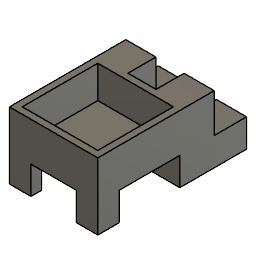
Pastillero (Autodesk Fusion 360 design; units mm, degrees)
Autodesk Fusion 360 part; units mm, degrees
sketch "Boceto1" plane through (0, 0, 0) normal (0, 1, 0) x (1, 0, 0)
  line L0 (-45, 25) -> (-4, 25)
  line L1 (-45, 25) -> (-45, -44)
  line L2 (-45, -44) -> (-4, -44)
  line L3 (-4, -44) -> (-4, 25)
  dimension "d1" = 41
  dimension "d2" = 69
  constraint horizontal L0
  constraint perpendicular L0 L1
  constraint perpendicular L1 L2
  constraint perpendicular L0 L3
  measures "d1" distance of L0.start L0.end
  measures "d2" distance of L0.start L1.end
extrude "Extruir1" add sketch "Boceto1" along normal blind 31
sketch "Boceto2" plane through (0, 31, 0) normal (0, 1, 0) x (-1, 0, 0)
  line L0 (45, -25) -> (45, 44)
  line L1 (45, 44) -> (4, 44)
  line L2 (4, 44) -> (4, -25)
  line L3 (4, -25) -> (45, -25)
  line L4 (42, 41) -> (42, 31.833)
  line L5 (42, 41) -> (7, 41)
  line L6 (7, 41) -> (7, 6)
  line L7 (7, 6) -> (42, 6)
  line L8 (42, 6) -> (42, 31.833)
  dimension "d7" = 35
  dimension "d8" = 35
  constraint perpendicular L4 L5
  constraint perpendicular L5 L6
  constraint perpendicular L6 L7
  constraint perpendicular L7 L8
  measures "d7" distance of L4.start L5.end
  measures "d8" distance of L5.end L6.end
extrude "Extruir2" cut sketch "Boceto2" against normal blind 15 contours L4 L5 L6 L7 L8
sketch "Boceto3" plane through (0, 0, 44) normal (0, 0, 1) x (1, 0, 0)
  line L0 (-45, 0) -> (-4, 0)
  line L1 (-4, 0) -> (-4, 31)
  line L2 (-4, 31) -> (-45, 31)
  line L3 (-45, 31) -> (-45, 0)
  line L4 (-45, 0) -> (-45, 13)
  line L5 (-45, 13) -> (-4, 13)
  line L6 (-4, 13) -> (-4, 0)
  dimension "d11" = 13
  constraint coincident L0.start L3.end
  constraint perpendicular L0 L4
  constraint coincident L1 L5.end
  constraint perpendicular L1 L5
  constraint coincident L0.end L1.start
  measures "d11" distance of L0.start L4.end
extrude "Extruir3" cut sketch "Boceto3" against normal blind 38 contours L0 L1 L3 L4 L5 L6
sketch "Boceto4" plane through (0, 31, 0) normal (0, 1, 0) x (-1, 0, 0)
  line L0 (7, 6) -> (7, 41)
  line L1 (7, 41) -> (42, 41)
  line L2 (42, 41) -> (42, 6)
  line L3 (42, 6) -> (7, 6)
  line L4 (45, -25) -> (45, 44)
  line L5 (45, 44) -> (4, 44)
  line L6 (4, 44) -> (4, -25)
  line L7 (4, -25) -> (45, -25)
  line L8 (31, -25) -> (18, -25)
  line L9 (31, -25) -> (31, 3)
  line L10 (31, 3) -> (18, 3)
  line L11 (18, 3) -> (18, -25)
  dimension "d14" = 14
  dimension "d15" = 13
  dimension "d16" = 28
  constraint parallel L7 L8
  constraint perpendicular L9 L10
  constraint perpendicular L8 L11
  measures "d14" distance of L4.start L8.start
  measures "d15" distance of L8.start L8.end
  measures "d16" distance of L8.start L9.end
extrude "Extruir4" cut sketch "Boceto4" against normal blind 28 contours L7 L8 L9 L10 L11
sketch "Boceto5" plane through (-45, 0, 0) normal (-1, 0, 0) x (0, 0, 1)
  line L0 (6, 0) -> (6, 13)
  line L1 (6, 13) -> (44, 13)
  line L2 (44, 13) -> (44, 31)
  line L3 (44, 31) -> (-25, 31)
  line L4 (-25, 31) -> (-25, 0)
  line L5 (-25, 0) -> (6, 0)
  line L6 (-25, 31) -> (-10, 31)
  line L7 (-10, 31) -> (-10, 13)
  line L8 (-10, 13) -> (-25, 13)
  line L9 (-25, 13) -> (-25, 31)
  dimension "d19" = 15
  dimension "d20" = 18
  constraint coincident L3.end L4.start
  constraint perpendicular L4 L6
  constraint perpendicular L6 L7
  constraint coincident L4 L8.end
  constraint perpendicular L4 L8
  measures "d19" distance of L3.end L6.end
  measures "d20" distance of L6.end L7.end
extrude "Extruir5" cut sketch "Boceto5" against normal blind 50 contours L3 L4 L6 L7 L8 L9
sketch "Boceto6" plane through (0, 0, 6) normal (0, 0, 1) x (1, 0, 0)
  line L0 (-45, 0) -> (-4, 0)
  line L1 (-4, 0) -> (-4, 13)
  line L2 (-4, 13) -> (-45, 13)
  line L3 (-45, 13) -> (-45, 0)
  line L4 (-31, 13) -> (-18, 13)
  line L5 (-18, 13) -> (-18, 3)
  line L6 (-18, 3) -> (-31, 3)
  line L7 (-31, 3) -> (-31, 13)
  dimension "d23" = 14
  dimension "d24" = 13
  dimension "d25" = 10
  constraint parallel L2 L4
  constraint perpendicular L4 L5
  constraint perpendicular L5 L6
  constraint perpendicular L4 L7
  measures "d23" distance of L2.end L4.start
  measures "d24" distance of L4.start L4.end
  measures "d25" distance of L4.end L5.end
extrude "Extruir6" cut sketch "Boceto6" against normal blind 30 contours L2 L4 L5 L6 L7
sketch "Boceto7" plane through (0, 0, 3) normal (0, 0, -1) x (-1, 0, 0)
  line L0 (18, 13) -> (31, 13)
  line L1 (31, 13) -> (31, 31)
  line L2 (31, 31) -> (18, 31)
  line L3 (18, 31) -> (18, 13)
  line L4 (18, 13) -> (31, 13)
  line L5 (31, 13) -> (31, 22.5)
  line L6 (31, 22.5) -> (18, 22.5)
  line L7 (18, 22.5) -> (18, 13)
  dimension "d28" = 9.5
  constraint coincident L0.start L3.end
  constraint coincident L0.end L1.start
  constraint perpendicular L4 L5
  constraint coincident L3 L6.end
  constraint perpendicular L3 L6
  measures "d28" distance of L0.end L5.end
extrude "Extruir7" add sketch "Boceto7" along normal blind 4.5 contours L0 L1 L3 L4 L5 L6 L7
sketch "Boceto8" plane through (0, 13, 0) normal (0, -1, 0) x (1, 0, 0)
  line L0 (-4, 44) -> (-45, 44)
  line L1 (-45, 44) -> (-45, 6)
  line L2 (-45, 6) -> (-31, 6)
  line L3 (-31, 6) -> (-31, -1.5)
  line L4 (-31, -1.5) -> (-18, -1.5)
  line L5 (-18, -1.5) -> (-18, 6)
  line L6 (-18, 6) -> (-4, 6)
  line L7 (-4, 6) -> (-4, 44)
  line L8 (-45, 44) -> (-35, 44)
  line L9 (-35, 44) -> (-35, 34)
  line L10 (-35, 34) -> (-45, 34)
  line L11 (-45, 34) -> (-45, 44)
  line L12 (-4, 44) -> (-14, 44)
  line L13 (-14, 44) -> (-14, 34)
  line L14 (-14, 34) -> (-4, 34)
  line L15 (-4, 34) -> (-4, 44)
  constraint horizontal L8
  constraint vertical L9
  constraint horizontal L10
  constraint vertical L11
  constraint coincident L0.end L1.start
  constraint horizontal L12
  constraint vertical L13
  constraint horizontal L14
  constraint vertical L15
  constraint coincident L0.start L7.end
extrude "Extruir8" add sketch "Boceto8" along normal blind 13 contours L0 L7 L12 L13 L14 L15 | L0 L1 L8 L9 L10 L11
sketch "Boceto9" plane through (0, 0, 0) normal (0, -1, 0) x (1, 0, 0)
  line L0 (-45, 34) -> (-35, 34)
  line L1 (-35, 34) -> (-35, 44)
  line L2 (-35, 44) -> (-45, 44)
  line L3 (-45, 44) -> (-45, 34)
  line L4 (-40, 34) -> (-40, 39)
  line L5 (-40, 39) -> (-35, 39)
  line L6 (-35, 34) -> (-40, 34)
  line L7 (-14, 34) -> (-9, 34)
  line L8 (-14, 34) -> (-14, 39)
  line L9 (-14, 39) -> (-9, 39)
  line L10 (-9, 39) -> (-9, 34)
  constraint midpoint L1 L5.end
  constraint midpoint L0 L4.start
  constraint perpendicular L0 L4
  constraint coincident L0.end L1.start
  constraint horizontal L7
  constraint perpendicular L7 L8
  constraint perpendicular L8 L9
  constraint perpendicular L7 L10
extrude "Extruir9" cut sketch "Boceto9" against normal blind 13 contours L0 L1 L4 L5 L6 | L7 L8 L9 L10
sketch "Boceto10" plane through (0, 22.5, 0) normal (0, 1, 0) x (-1, 0, 0)
  line L0 (31, 3) -> (18, 3)
  line L1 (18, 3) -> (18, -1.5)
  line L2 (18, -1.5) -> (31, -1.5)
  line L3 (31, -1.5) -> (31, 3)
  circle A0 centre (24.5, 0.75) radius 0.5
  dimension "d35" = 1
  measures "d35" diameter of A0
extrude "Extruir10" cut sketch "Boceto10" against normal blind 4 contours A0
extrude "Extruir11" add 1 faces at (-22.3333, 3, -14.6667) along direction (0, 1, 0) blind 3
extrude "Extruir12" cut 1 faces at (-22.3333, 6, -14.6667) along direction (0, -1, 0) blind 3
extrude "Extruir13" cut 1 faces at (-29, 22.5, 0.75) along direction (0, -1, 0) blind 3
extrude "Extruir14" cut 1 faces at (-24.1479, 18.5, 0.7889) along direction (0, -1, 0) blind 3
